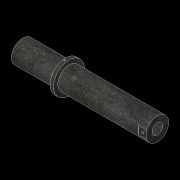
# Autodesk Inventor part: KON_Nietmaschine_Dorn
Saved by Autodesk Inventor 2019 (Build 230136000, 136)
## iProperties
Created: 2021-12-29
Part Number: KON_Nietmaschine_Dorn
Material: Stahl
Document SubType Name: Modeling
Designer: Jonas Nebl
Density: 7.85 g/cm^3
Appearance: Platte
Mass: 1208.26 g
Surface Area: 231.998 cm^2
Volume: 153.918 cm^3
Author: Jonas Nebl
Autodesk Inventor part; units mm, degrees
ref_plane "YZ Plane" through (0, 0, 0) normal (1, 0, 0) x (0, 1, 0)
sketch "Skizze1" plane through (0, 0, 0) normal (0, 0, 1) x (1, 0, 0)
  line L0 (-95.375, 0) -> (-95.375, -16)
  line L1 (-95.375, -16) -> (-34.625, -16)
  line L2 (-34.625, -16) -> (-34.625, -22)
  line L3 (-34.625, -22) -> (-29.625, -22)
  line L4 (-29.625, -22) -> (-29.625, -16)
  line L5 (-29.625, -16) -> (95.375, -16)
  line L6 (95.375, -16) -> (95.375, 0)
  line L7 (0, -26.4) -> (0, 4.4) projected
  line L8 (-95.375, 0) -> (95.375, 0)
  point P0 (0, 0)
  dimension "d0" = 190.75
  dimension "d1" = 60.75
  dimension "d2" = 5
  dimension "d3" = 44
  dimension "d4" = 32
  constraints: 16 end point, 4 horizontal, 3 vertical, 1 midpoint, 1 point on line, 1 other
  measures "d0" distance of L0.start L6.end
  measures "d1" distance of L0.end L1.end
  measures "d2" distance of L2.end L3.end
  measures "d3" diameter of L3 L8
  measures "d4" diameter of L1 L8
revolve "Umdrehung1" add sketch "Skizze1" angle 360 about axis through (-95.375, 0, 0) along (1, 0, 0)
sketch "Skizze2" plane through (95.375, 0, 0) normal (1, 0, 0) x (0, 0, -1)
  point P0 (0, 0)
  point P1 (0, 0)
  constraints: 1 coincident
hole "Bohrung1" at (95.375, 0, 0) direction (-1, 0, 0) diameter 15 depth 15 tip angle 118
ref_plane "Arbeitsebene1" through (0, 0, 17) normal (0, 0, 1) x (1, 0, 0)
sketch "Skizze3" plane through (0, 0, 17) normal (0, 0, 1) x (1, 0, 0)
  line L0 (95.375, 16) -> (95.375, -16) projected
  line L1 (-19.1, 0) -> (114.6, 0) projected
  point P0 (0, 0)
  point P1 (89.375, 0)
  dimension "d14" = 6
  constraints: 1 point on line
  measures "d14" distance from line of L0 point (89.375, 0)
hole "Bohrung2" at (89.375, 0, 17) direction (0, 0, -1) diameter 3.3 depth 15 tip angle 118
thread "Gewinde1" size "M4x0.7" class "6H" standard "ANSI Metric M Profile" full length
ref_plane "Arbeitsebene2" through (32.875, 16, 0) normal (0, 1, 0) x (-1, 0, 0)
sketch "Skizze4" plane through (32.875, 16, 0) normal (0, 1, 0) x (-1, 0, 0)
  line L0 (-51.236, 14.9255) -> (-64.8567, 14.9255)
  line L1 (-64.8567, 14.9255) -> (-64.8567, 17.1103)
  line L2 (-64.8567, 17.1103) -> (-51.236, 17.1103)
  line L3 (-51.236, 17.1103) -> (-51.236, 14.9255)
  point P0 (32.875, 0)
  constraints: 8 end point, 2 parallel, 1 horizontal, 1 perpendicular
extrude "Extrusion1" cut sketch "Skizze4" against normal through all
